Autodesk Inventor part; units mm, degrees
(part 2 of 3)
sketch "Sketch8" plane through (-4.2986, 24.5, 27.7) normal (0, 1, 0) x (1, 0, 0)
  circle A0 centre (15.7486, 17.6859) radius 1.25 projected
  arc A1 (23.4169, 15.4064) -> (22.432, 16.0745) centre (20.1359, 11.63) ccw projected
  arc A2 (22.432, 16.0745) -> (22.5072, 16.4265) centre (15.7486, 17.6859) ccw projected
  arc A3 (22.5072, 16.4265) -> (23.6791, 16.634) centre (22.2271, 21.4212) ccw projected
  arc A4 (23.6791, 16.634) -> (23.7233, 17.0505) centre (15.7486, 17.6859) ccw projected
  arc A5 (23.7233, 17.0505) -> (22.621, 17.4993) centre (21.2992, 12.6745) ccw projected
  arc A6 (22.621, 17.4993) -> (22.6214, 17.8592) centre (15.7486, 17.6859) ccw projected
  arc A7 (22.6214, 17.8592) -> (23.7245, 18.3059) centre (21.3089, 22.6865) ccw projected
  arc A8 (23.7245, 18.3059) -> (23.6811, 18.7224) centre (15.7486, 17.6859) ccw projected
  arc A9 (23.6811, 18.7224) -> (22.5097, 18.9322) centre (22.2198, 13.9381) ccw projected
  arc A10 (22.5097, 18.9322) -> (22.4352, 19.2844) centre (15.7486, 17.6859) ccw projected
  arc A11 (22.4352, 19.2844) -> (23.4213, 19.9506) centre (20.1477, 23.7333) ccw projected
  arc A12 (23.4213, 19.9506) -> (23.2923, 20.3491) centre (15.7486, 17.6859) ccw projected
  arc A13 (23.2923, 20.3491) -> (22.1028, 20.3107) centre (22.8576, 15.3654) ccw projected
  arc A14 (22.1028, 20.3107) -> (21.9567, 20.6397) centre (15.7486, 17.6859) ccw projected
  arc A15 (21.9567, 20.6397) -> (22.7828, 21.4964) centre (18.7942, 24.5158) ccw projected
  arc A16 (22.7828, 21.4964) -> (22.5737, 21.8593) centre (15.7486, 17.6859) ccw projected
  arc A17 (22.5737, 21.8593) -> (21.4182, 21.5745) centre (23.1847, 16.8942) ccw projected
  arc A18 (21.4182, 21.5745) -> (21.2069, 21.8659) centre (15.7486, 17.6859) ccw projected
  arc A19 (21.2069, 21.8659) -> (21.8368, 22.8756) centre (17.3077, 24.9998) ccw projected
  arc A20 (21.8368, 22.8756) -> (21.5569, 23.1871) centre (15.7486, 17.6859) ccw projected
  arc A21 (21.5569, 23.1871) -> (20.4858, 22.6683) centre (23.1868, 18.4576) ccw projected
  arc A22 (20.4858, 22.6683) -> (20.2186, 22.9094) centre (15.7486, 17.6859) ccw projected
  arc A23 (20.2186, 22.9094) -> (20.6248, 24.028) centre (15.753, 25.1641) ccw projected
  arc A24 (20.6248, 24.028) -> (20.2862, 24.2745) centre (15.7486, 17.6859) ccw projected
  arc A25 (20.2862, 24.2745) -> (19.3464, 23.5443) centre (22.8638, 19.9872) ccw projected
  arc A26 (19.3464, 23.5443) -> (19.0349, 23.7246) centre (15.7486, 17.6859) ccw projected
  arc A27 (19.0349, 23.7246) -> (19.1997, 24.9033) centre (14.1981, 25.0016) ccw projected
  arc A28 (19.1997, 24.9033) -> (18.8172, 25.074) centre (15.7486, 17.6859) ccw projected
  arc A29 (18.8172, 25.074) -> (18.0498, 24.1644) centre (22.2299, 21.4163) ccw projected
  arc A30 (18.0498, 24.1644) -> (17.7076, 24.2759) centre (15.7486, 17.6859) ccw projected
  arc A31 (17.7076, 24.2759) -> (17.6237, 25.4631) centre (12.711, 24.5194) ccw projected
  arc A32 (17.6237, 25.4631) -> (17.2141, 25.5505) centre (15.7486, 17.6859) ccw projected
  arc A33 (17.2141, 25.5505) -> (16.6525, 24.5012) centre (21.3127, 22.6823) ccw projected
  arc A34 (16.6525, 24.5012) -> (16.2946, 24.5392) centre (15.7486, 17.6859) ccw projected
  arc A35 (16.2946, 24.5392) -> (15.9657, 25.683) centre (11.3566, 23.7385) ccw projected
  arc A36 (15.9657, 25.683) -> (15.5469, 25.6834) centre (15.7486, 17.6859) ccw projected
  arc A37 (15.5469, 25.6834) -> (15.2158, 24.5402) centre (20.1523, 23.7299) ccw projected
  arc A38 (15.2158, 24.5402) -> (14.8578, 24.503) centre (15.7486, 17.6859) ccw projected
  arc A39 (14.8578, 24.503) -> (14.2983, 25.5534) centre (10.1942, 22.6931) ccw projected
  arc A40 (14.2983, 25.5534) -> (13.8885, 25.4667) centre (15.7486, 17.6859) ccw projected
  arc A41 (13.8885, 25.4667) -> (13.8024, 24.2797) centre (18.7994, 24.5135) ccw projected
  arc A42 (13.8024, 24.2797) -> (13.4599, 24.1688) centre (15.7486, 17.6859) ccw projected
  arc A43 (13.4599, 24.1688) -> (12.6943, 25.0799) centre (9.2745, 21.4288) ccw projected
  arc A44 (12.6943, 25.0799) -> (12.3115, 24.9099) centre (15.7486, 17.6859) ccw projected
  arc A45 (12.3115, 24.9099) -> (12.474, 23.731) centre (17.3132, 24.9986) ccw projected
  arc A46 (12.474, 23.731) -> (12.1621, 23.5513) centre (15.7486, 17.6859) ccw projected
  arc A47 (12.1621, 23.5513) -> (11.2237, 24.2833) centre (8.6378, 20.001) ccw projected
  arc A48 (11.2237, 24.2833) -> (10.8846, 24.0375) centre (15.7486, 17.6859) ccw projected
  arc A49 (10.8846, 24.0375) -> (11.2887, 22.918) centre (15.7587, 25.1641) ccw projected
  arc A50 (11.2887, 22.918) -> (11.021, 22.6775) centre (15.7486, 17.6859) ccw projected
  arc A51 (11.021, 22.6775) -> (9.9509, 23.1984) centre (8.3118, 18.472) ccw projected
  arc A52 (9.9509, 23.1984) -> (9.6704, 22.8874) centre (15.7486, 17.6859) ccw projected
  arc A53 (9.6704, 22.8874) -> (10.2983, 21.8764) centre (14.2036, 25.0028) ccw projected
  arc A54 (10.2983, 21.8764) -> (10.0865, 21.5855) centre (15.7486, 17.6859) ccw projected
  arc A55 (10.0865, 21.5855) -> (8.9315, 21.8725) centre (8.3109, 16.9086) ccw projected
  arc A56 (8.9315, 21.8725) -> (8.7217, 21.51) centre (15.7486, 17.6859) ccw projected
  arc A57 (8.7217, 21.51) -> (9.5462, 20.6517) centre (12.7161, 24.5217) ccw projected
  arc A58 (9.5462, 20.6517) -> (9.3994, 20.323) centre (15.7486, 17.6859) ccw projected
  arc A59 (9.3994, 20.323) -> (8.21, 20.3637) centre (8.635, 15.3792) ccw projected
  arc A60 (8.21, 20.3637) -> (8.0802, 19.9655) centre (15.7486, 17.6859) ccw projected
  arc A61 (8.0802, 19.9655) -> (9.0651, 19.2973) centre (11.3612, 23.7418) ccw projected
  arc A62 (9.0651, 19.2973) -> (8.9899, 18.9453) centre (15.7486, 17.6859) ccw projected
  arc A63 (8.9899, 18.9453) -> (7.818, 18.7378) centre (9.2701, 13.9507) ccw projected
  arc A64 (7.818, 18.7378) -> (7.7738, 18.3213) centre (15.7486, 17.6859) ccw projected
  arc A65 (7.7738, 18.3213) -> (8.8761, 17.8726) centre (10.198, 22.6973) ccw projected
  arc A66 (8.8761, 17.8726) -> (8.8757, 17.5126) centre (15.7486, 17.6859) ccw projected
  arc A67 (8.8757, 17.5126) -> (7.7726, 17.066) centre (10.1882, 12.6853) ccw projected
  arc A68 (7.7726, 17.066) -> (7.816, 16.6494) centre (15.7486, 17.6859) ccw projected
  arc A69 (7.816, 16.6494) -> (8.9875, 16.4396) centre (9.2773, 21.4337) ccw projected
  arc A70 (8.9875, 16.4396) -> (9.062, 16.0875) centre (15.7486, 17.6859) ccw projected
  arc A71 (9.062, 16.0875) -> (8.0758, 15.4212) centre (11.3494, 11.6386) ccw projected
  arc A72 (8.0758, 15.4212) -> (8.2048, 15.0228) centre (15.7486, 17.6859) ccw projected
  arc A73 (8.2048, 15.0228) -> (9.3943, 15.0611) centre (8.6395, 20.0064) ccw projected
  arc A74 (9.3943, 15.0611) -> (9.5404, 14.7322) centre (15.7486, 17.6859) ccw projected
  arc A75 (9.5404, 14.7322) -> (8.7143, 13.8755) centre (12.7029, 10.8561) ccw projected
  arc A76 (8.7143, 13.8755) -> (8.9234, 13.5126) centre (15.7486, 17.6859) ccw projected
  arc A77 (8.9234, 13.5126) -> (10.0789, 13.7974) centre (8.3124, 18.4776) ccw projected
  arc A78 (10.0789, 13.7974) -> (10.2902, 13.506) centre (15.7486, 17.6859) ccw projected
  arc A79 (10.2902, 13.506) -> (9.6603, 12.4962) centre (14.1894, 10.3721) ccw projected
  arc A80 (9.6603, 12.4962) -> (9.9402, 12.1847) centre (15.7486, 17.6859) ccw projected
  arc A81 (9.9402, 12.1847) -> (11.0113, 12.7036) centre (8.3103, 16.9143) ccw projected
  arc A82 (11.0113, 12.7036) -> (11.2785, 12.4625) centre (15.7486, 17.6859) ccw projected
  arc A83 (11.2785, 12.4625) -> (10.8723, 11.3438) centre (15.7441, 10.2078) ccw projected
  arc A84 (10.8723, 11.3438) -> (11.2109, 11.0973) centre (15.7486, 17.6859) ccw projected
  arc A85 (11.2109, 11.0973) -> (12.1507, 11.8275) centre (8.6333, 15.3846) ccw projected
  arc A86 (12.1507, 11.8275) -> (12.4622, 11.6472) centre (15.7486, 17.6859) ccw projected
  arc A87 (12.4622, 11.6472) -> (12.2975, 10.4686) centre (17.299, 10.3702) ccw projected
  arc A88 (12.2975, 10.4686) -> (12.6799, 10.2979) centre (15.7486, 17.6859) ccw projected
  arc A89 (12.6799, 10.2979) -> (13.4474, 11.2075) centre (9.2672, 13.9556) ccw projected
  arc A90 (13.4474, 11.2075) -> (13.7896, 11.0959) centre (15.7486, 17.6859) ccw projected
  arc A91 (13.7896, 11.0959) -> (13.8735, 9.9088) centre (18.7862, 10.8525) ccw projected
  arc A92 (13.8735, 9.9088) -> (14.283, 9.8213) centre (15.7486, 17.6859) ccw projected
  arc A93 (14.283, 9.8213) -> (14.8446, 10.8706) centre (10.1844, 12.6896) ccw projected
  arc A94 (14.8446, 10.8706) -> (15.2025, 10.8326) centre (15.7486, 17.6859) ccw projected
  arc A95 (15.2025, 10.8326) -> (15.5314, 9.6889) centre (20.1405, 11.6334) ccw projected
  arc A96 (15.5314, 9.6889) -> (15.9502, 9.6885) centre (15.7486, 17.6859) ccw projected
  arc A97 (15.9502, 9.6885) -> (16.2813, 10.8316) centre (11.3448, 11.6419) ccw projected
  arc A98 (16.2813, 10.8316) -> (16.6393, 10.8689) centre (15.7486, 17.6859) ccw projected
  arc A99 (16.6393, 10.8689) -> (17.1988, 9.8185) centre (21.303, 12.6788) ccw projected
  arc A100 (17.1988, 9.8185) -> (17.6086, 9.9052) centre (15.7486, 17.6859) ccw projected
  arc A101 (17.6086, 9.9052) -> (17.6948, 11.0921) centre (12.6977, 10.8584) ccw projected
  arc A102 (17.6948, 11.0921) -> (18.0372, 11.203) centre (15.7486, 17.6859) ccw projected
  arc A103 (18.0372, 11.203) -> (18.8029, 10.2919) centre (22.2226, 13.943) ccw projected
  arc A104 (18.8029, 10.2919) -> (19.1856, 10.4619) centre (15.7486, 17.6859) ccw projected
  arc A105 (19.1856, 10.4619) -> (19.0232, 11.6409) centre (14.1839, 10.3733) ccw projected
  arc A106 (19.0232, 11.6409) -> (19.335, 11.8205) centre (15.7486, 17.6859) ccw projected
  arc A107 (19.335, 11.8205) -> (20.2734, 11.0885) centre (22.8594, 15.3708) ccw projected
  arc A108 (20.2734, 11.0885) -> (20.6125, 11.3344) centre (15.7486, 17.6859) ccw projected
  arc A109 (20.6125, 11.3344) -> (20.2084, 12.4538) centre (15.7385, 10.2078) ccw projected
  arc A110 (20.2084, 12.4538) -> (20.4762, 12.6944) centre (15.7486, 17.6859) ccw projected
  arc A111 (20.4762, 12.6944) -> (21.5462, 12.1735) centre (23.1853, 16.8998) ccw projected
  arc A112 (21.5462, 12.1735) -> (21.8268, 12.4844) centre (15.7486, 17.6859) ccw projected
  arc A113 (21.8268, 12.4844) -> (21.1988, 13.4954) centre (17.2935, 10.3691) ccw projected
  arc A114 (21.1988, 13.4954) -> (21.4106, 13.7864) centre (15.7486, 17.6859) ccw projected
  arc A115 (21.4106, 13.7864) -> (22.5656, 13.4993) centre (23.1862, 18.4632) ccw projected
  arc A116 (22.5656, 13.4993) -> (22.7754, 13.8618) centre (15.7486, 17.6859) ccw projected
  arc A117 (22.7754, 13.8618) -> (21.951, 14.7201) centre (18.781, 10.8502) ccw projected
  arc A118 (21.951, 14.7201) -> (22.0977, 15.0488) centre (15.7486, 17.6859) ccw projected
  arc A119 (22.0977, 15.0488) -> (23.2871, 15.0081) centre (22.8621, 19.9926) ccw projected
  arc A120 (23.2871, 15.0081) -> (23.4169, 15.4064) centre (15.7486, 17.6859) ccw projected
  circle A121 centre (15.7486, 17.6859) radius 8
  circle A122 centre (15.7486, 17.6859) radius 8.4
  line L0 (7.6044, 15.6287) -> (7.3834, 15.5214)
  line L1 (31.7444, 20.1683) -> (32.1777, 20.1683) projected
  line L2 (32.1777, 20.1683) -> (35.8615, 24.6355) projected
  line L3 (39.4105, 21.7089) -> (39.4105, 0) projected
  line L4 (39.4105, 0) -> (43.7986, 0) projected
  line L5 (43.7986, 0) -> (43.7986, 27.7) projected
  line L6 (43.7986, 27.7) -> (-10.0014, 27.7) projected
  line L7 (-10.0014, 27.7) -> (-10.0014, 0) projected
  line L8 (-10.0014, 0) -> (0, 0) projected
  arc A123 (0, 0) -> (10.1832, 0) centre (5.0916, 5.5748) ccw projected
  line L9 (10.1832, 0) -> (23.789, 0) projected
  arc A124 (20.8845, 2.8543) -> (23.789, 1) centre (29.9486, 13.85) ccw projected
  line L10 (20.8845, 2.8543) -> (20.8845, 5.5354) projected
  line L11 (24.1705, 10.4583) -> (24.5486, 13.85) projected
  arc A125 (31.7444, 20.1683) -> (27.6265, 18.7253) centre (28.4986, 22.8337) ccw projected
  line L12 (39.4105, 21.7089) -> (39.4105, 0) projected
  line L13 (10.1832, 0) -> (23.789, 0) projected
  line L14 (39.4105, 0) -> (23.789, 0)
  circle A126 centre (28.4986, 22.8337) radius 4.2
  line L15 (23.789, 0) -> (23.789, 1) projected
  arc A127 (20.8845, 5.5354) -> (24.0356, 3.0645) centre (29.9486, 13.85) ccw projected
  line L16 (24.0356, 3.0645) -> (27.7194, 7.5317) projected
  arc A128 (39.4105, 21.7089) -> (35.8615, 24.6355) centre (29.9486, 13.85) ccw projected
  arc A129 (24.1705, 10.4583) -> (27.7194, 7.5317) centre (29.9486, 13.85) ccw projected
  arc A130 (27.6265, 18.7253) -> (24.5486, 13.85) centre (29.9486, 13.85) ccw projected
  point P0 (4.2986, 27.7)
  dimension "d38" = 0.4
  constraints: 4 end point, 2 coincident, 9 other
extrude "Extrusion8" add sketch "Sketch8" along normal blind 2.1 contours A0 | A120 A119 A118 A117 A116 A115 A114 A113 A112 A111 A110 A109 A108 A107 A106 A105 A104 A103 A102 A101 A100 A99 A98 A97 A96 A95 A94 A93 A92 A91 A90 A89 A88 A87 A86 A85 A84 A83 A82 A81 A80 A79 A78 A77 A76 A75 A74 A73 A72 A71 A70 A69 A68 A67 A66 A65 A64 A63 A62 A61 A60 A59 A58 A57 A56 A55 A54 A53 A52 A51 A50 A49 A48 A47 A46 A45 A44 A43 A42 A41 A40 A39 A38 A37 A36 A35 A34 A33 A32 A31 A30 A29 A28 A27 A26 A25 A24 A23 A22 A21 A20 A19 A18 A17 A16 A15 A14 A13 A12 A11 A10 A9 A8 A7 A6 A5 A4 A3 A2 A1 | A1 A2 A3 A121 | A121 A117 A118 A119 | A5 A6 A7 A121 | A121 A113 A114 A115 | A121 A109 A110 A111 | A9 A10 A11 A121 | A121 A105 A106 A107 | A13 A14 A15 A121 | A121 A101 A102 A103 | A17 A18 A19 A121 | A121 A97 A98 A99 | A21 A22 A23 A121 | A121 A93 A94 A95 | A25 A26 A27 A121 | A121 A89 A90 A91 | A29 A30 A31 A121 | A121 A85 A86 A87 | A33 A34 A35 A121 | A121 A81 A82 A83 | A37 A38 A39 A121 | A121 A77 A78 A79 | A41 A42 A43 A121 | A121 A73 A74 A75 | A45 A46 A47 A121 | A121 A69 A70 A71 | A49 A50 A51 A121 | A121 A65 A66 A67 | A53 A54 A55 A121 | A121 A61 A62 A63 | A57 A58 A59 A121 | A122 | A125 A130 L11 A129 L16 A127 L10 A124 L15 L9 A123 L8 L7 L6 L5 L4 L3 A128 L2 L1 | L1 L2 A128 L3 L14 L15 A124 L10 A127 L16 A129 L11 A130 A126
sketch "Sketch10" plane through (-4.2986, 26.6, 27.7) normal (0, 1, 0) x (1, 0, 0)
  line L0 (36.5978, 20.9908) -> (36.5978, 20.9908)
  line L1 (36.5978, 20.9908) -> (36.5978, 20.9908)
  line L2 (43.7986, 0) -> (43.7986, 27.7) projected
  line L3 (43.7986, 0) -> (-14.5322, 0)
  line L4 (43.7986, 0) -> (43.7986, 27.7) projected
  line L5 (43.7986, 27.7) -> (-10.0014, 27.7) projected
  line L6 (-10.0014, 27.7) -> (-10.0014, 0) projected
  line L7 (-10.0014, 0) -> (0, 0) projected
  arc A0 (0, 0) -> (10.1832, 0) centre (5.0916, 5.5748) ccw projected
  circle A1 centre (28.4986, 22.8337) radius 5.5 projected
  circle A2 centre (2.9986, 22.8337) radius 5.5 projected
  circle A3 centre (28.4986, 22.8337) radius 5.9
  circle A4 centre (2.9986, 22.8337) radius 5.9
  line L8 (10.1832, 0) -> (43.7986, 0) projected
  point P0 (4.2986, 27.7)
  dimension "d63" = 0.4
  dimension "d64" = 0.4
  constraints: 6 end point, 3 horizontal, 2 centre point
  measures "d63" radial gap between concentric circles of A1 A3
  measures "d64" radial gap between concentric circles of A2 A4
extrude "Extrusion10" cut sketch "Sketch10" against normal blind 1 contours A3 L5 A1 | L5 A1 A3 | A1 L5 | L5 A1 | A4 L5 A2 | L5 A2 A4 | A2 L5 | L5 A2
sketch "Sketch11" plane through (-4.2986, 25.6, 27.7) normal (0, 1, 0) x (1, 0, 0)
  circle A0 centre (28.4986, 22.8337) radius 3 projected
  arc A1 (18.0491, 21.8046) -> (19.212, 21.5492) centre (19.8204, 27.0964) ccw projected
  arc A2 (19.212, 21.5492) -> (19.2696, 21.1856) centre (28.4986, 22.8337) ccw projected
  arc A3 (19.2696, 21.1856) -> (18.2425, 20.5835) centre (21.5624, 16.098) ccw projected
  arc A4 (18.2425, 20.5835) -> (18.3388, 20.1826) centre (28.4986, 22.8337) ccw projected
  arc A5 (18.3388, 20.1826) -> (19.5272, 20.1123) centre (19.2604, 25.6863) ccw projected
  arc A6 (19.5272, 20.1123) -> (19.641, 19.7622) centre (28.4986, 22.8337) ccw projected
  arc A7 (19.641, 19.7622) -> (18.7208, 19.0068) centre (22.7015, 15.0959) ccw projected
  arc A8 (18.7208, 19.0068) -> (18.8786, 18.6259) centre (28.4986, 22.8337) ccw projected
  arc A9 (18.8786, 18.6259) -> (20.0634, 18.7424) centre (18.9279, 24.2061) ccw projected
  arc A10 (20.0634, 18.7424) -> (20.2305, 18.4144) centre (28.4986, 22.8337) ccw projected
  arc A11 (20.2305, 18.4144) -> (19.4399, 17.5243) centre (23.9833, 14.2843) ccw projected
  arc A12 (19.4399, 17.5243) -> (19.6553, 17.1728) centre (28.4986, 22.8337) ccw projected
  arc A13 (19.6553, 17.1728) -> (20.8073, 17.4732) centre (18.8311, 22.692) ccw projected
  arc A14 (20.8073, 17.4732) -> (21.0237, 17.1754) centre (28.4986, 22.8337) ccw projected
  arc A15 (21.0237, 17.1754) -> (20.382, 16.1726) centre (25.3763, 13.6832) ccw projected
  arc A16 (20.382, 16.1726) -> (20.6497, 15.8591) centre (28.4986, 22.8337) ccw projected
  arc A17 (20.6497, 15.8591) -> (21.7406, 16.336) centre (18.9723, 21.1814) ccw projected
  arc A18 (21.7406, 16.336) -> (22.0009, 16.0757) centre (28.4986, 22.8337) ccw projected
  arc A19 (22.0009, 16.0757) -> (21.5239, 14.9849) centre (26.8462, 13.3075) ccw projected
  arc A20 (21.5239, 14.9849) -> (21.8374, 14.7171) centre (28.4986, 22.8337) ccw projected
  arc A21 (21.8374, 14.7171) -> (22.8402, 15.3589) centre (19.3481, 19.7115) ccw projected
  arc A22 (22.8402, 15.3589) -> (23.138, 15.1425) centre (28.4986, 22.8337) ccw projected
  arc A23 (23.138, 15.1425) -> (22.8376, 13.9905) centre (28.3568, 13.1663) ccw projected
  arc A24 (22.8376, 13.9905) -> (23.1892, 13.775) centre (28.4986, 22.8337) ccw projected
  arc A25 (23.1892, 13.775) -> (24.0792, 14.5657) centre (19.9491, 18.3185) ccw projected
  arc A26 (24.0792, 14.5657) -> (24.4072, 14.3986) centre (28.4986, 22.8337) ccw projected
  arc A27 (24.4072, 14.3986) -> (24.2907, 13.2138) centre (29.8709, 13.2631) ccw projected
  arc A28 (24.2907, 13.2138) -> (24.6716, 13.056) centre (28.4986, 22.8337) ccw projected
  arc A29 (24.6716, 13.056) -> (25.427, 13.9762) centre (20.7607, 17.0367) ccw projected
  arc A30 (25.427, 13.9762) -> (25.7771, 13.8624) centre (28.4986, 22.8337) ccw projected
  arc A31 (25.7771, 13.8624) -> (25.8474, 12.6739) centre (31.3512, 13.5956) ccw projected
  arc A32 (25.8474, 12.6739) -> (26.2483, 12.5777) centre (28.4986, 22.8337) ccw projected
  arc A33 (26.2483, 12.5777) -> (26.8505, 13.6047) centre (21.7629, 15.8976) ccw projected
  arc A34 (26.8505, 13.6047) -> (27.2141, 13.5471) centre (28.4986, 22.8337) ccw projected
  arc A35 (27.2141, 13.5471) -> (27.4694, 12.3843) centre (32.7612, 14.1556) ccw projected
  arc A36 (27.4694, 12.3843) -> (27.8804, 12.3519) centre (28.4986, 22.8337) ccw projected
  arc A37 (27.8804, 12.3519) -> (28.3145, 13.4605) centre (22.9308, 14.9293) ccw projected
  arc A38 (28.3145, 13.4605) -> (28.6826, 13.4605) centre (28.4986, 22.8337) ccw projected
  arc A39 (28.6826, 13.4605) -> (29.1167, 12.3519) centre (34.0663, 14.9293) ccw projected
  arc A40 (29.1167, 12.3519) -> (29.5277, 12.3843) centre (28.4986, 22.8337) ccw projected
  arc A41 (29.5277, 12.3843) -> (29.7831, 13.5471) centre (24.2359, 14.1556) ccw projected
  arc A42 (29.7831, 13.5471) -> (30.1467, 13.6047) centre (28.4986, 22.8337) ccw projected
  arc A43 (30.1467, 13.6047) -> (30.7488, 12.5777) centre (35.2343, 15.8976) ccw projected
  arc A44 (30.7488, 12.5777) -> (31.1497, 12.6739) centre (28.4986, 22.8337) ccw projected
  arc A45 (31.1497, 12.6739) -> (31.22, 13.8624) centre (25.646, 13.5956) ccw projected
  arc A46 (31.22, 13.8624) -> (31.5701, 13.9762) centre (28.4986, 22.8337) ccw projected
  arc A47 (31.5701, 13.9762) -> (32.3255, 13.056) centre (36.2364, 17.0367) ccw projected
  arc A48 (32.3255, 13.056) -> (32.7064, 13.2138) centre (28.4986, 22.8337) ccw projected
  arc A49 (32.7064, 13.2138) -> (32.5899, 14.3986) centre (27.1262, 13.2631) ccw projected
  arc A50 (32.5899, 14.3986) -> (32.9179, 14.5657) centre (28.4986, 22.8337) ccw projected
  arc A51 (32.9179, 14.5657) -> (33.808, 13.775) centre (37.048, 18.3185) ccw projected
  arc A52 (33.808, 13.775) -> (34.1595, 13.9905) centre (28.4986, 22.8337) ccw projected
  arc A53 (34.1595, 13.9905) -> (33.8591, 15.1425) centre (28.6403, 13.1663) ccw projected
  arc A54 (33.8591, 15.1425) -> (34.1569, 15.3589) centre (28.4986, 22.8337) ccw projected
  arc A55 (34.1569, 15.3589) -> (35.1597, 14.7171) centre (37.6491, 19.7115) ccw projected
  arc A56 (35.1597, 14.7171) -> (35.4732, 14.9849) centre (28.4986, 22.8337) ccw projected
  arc A57 (35.4732, 14.9849) -> (34.9963, 16.0757) centre (30.1509, 13.3075) ccw projected
  arc A58 (34.9963, 16.0757) -> (35.2566, 16.336) centre (28.4986, 22.8337) ccw projected
  arc A59 (35.2566, 16.336) -> (36.3474, 15.8591) centre (38.0248, 21.1814) ccw projected
  arc A60 (36.3474, 15.8591) -> (36.6152, 16.1726) centre (28.4986, 22.8337) ccw projected
  arc A61 (36.6152, 16.1726) -> (35.9734, 17.1754) centre (31.6208, 13.6832) ccw projected
  arc A62 (35.9734, 17.1754) -> (36.1898, 17.4732) centre (28.4986, 22.8337) ccw projected
  arc A63 (36.1898, 17.4732) -> (37.3418, 17.1728) centre (38.166, 22.692) ccw projected
  arc A64 (37.3418, 17.1728) -> (37.5573, 17.5243) centre (28.4986, 22.8337) ccw projected
  arc A65 (37.5573, 17.5243) -> (36.7666, 18.4144) centre (33.0138, 14.2843) ccw projected
  arc A66 (36.7666, 18.4144) -> (36.9337, 18.7424) centre (28.4986, 22.8337) ccw projected
  arc A67 (36.9337, 18.7424) -> (38.1185, 18.6259) centre (38.0692, 24.2061) ccw projected
  arc A68 (38.1185, 18.6259) -> (38.2763, 19.0068) centre (28.4986, 22.8337) ccw projected
  arc A69 (38.2763, 19.0068) -> (37.3561, 19.7622) centre (34.2956, 15.0959) ccw projected
  arc A70 (37.3561, 19.7622) -> (37.4699, 20.1123) centre (28.4986, 22.8337) ccw projected
  arc A71 (37.4699, 20.1123) -> (38.6584, 20.1826) centre (37.7367, 25.6863) ccw projected
  arc A72 (38.6584, 20.1826) -> (38.7546, 20.5835) centre (28.4986, 22.8337) ccw projected
  arc A73 (38.7546, 20.5835) -> (37.7276, 21.1856) centre (35.4347, 16.098) ccw projected
  arc A74 (37.7276, 21.1856) -> (37.7851, 21.5492) centre (28.4986, 22.8337) ccw projected
  arc A75 (37.7851, 21.5492) -> (38.948, 21.8046) centre (37.1767, 27.0964) ccw projected
  arc A76 (38.948, 21.8046) -> (38.9804, 22.2156) centre (28.4986, 22.8337) ccw projected
  arc A77 (38.9804, 22.2156) -> (37.8718, 22.6497) centre (36.403, 17.266) ccw projected
  arc A78 (37.8718, 22.6497) -> (37.8718, 23.0178) centre (28.4986, 22.8337) ccw projected
  arc A79 (37.8718, 23.0178) -> (38.9804, 23.4519) centre (36.403, 28.4015) ccw projected
  arc A80 (38.9804, 23.4519) -> (38.948, 23.8629) centre (28.4986, 22.8337) ccw projected
  arc A81 (38.948, 23.8629) -> (37.7851, 24.1182) centre (37.1767, 18.5711) ccw projected
  arc A82 (37.7851, 24.1182) -> (37.7276, 24.4818) centre (28.4986, 22.8337) ccw projected
  arc A83 (37.7276, 24.4818) -> (38.7546, 25.084) centre (35.4347, 29.5694) ccw projected
  arc A84 (38.7546, 25.084) -> (38.6584, 25.4849) centre (28.4986, 22.8337) ccw projected
  arc A85 (38.6584, 25.4849) -> (37.4699, 25.5552) centre (37.7367, 19.9811) ccw projected
  arc A86 (37.4699, 25.5552) -> (37.3561, 25.9053) centre (28.4986, 22.8337) ccw projected
  arc A87 (37.3561, 25.9053) -> (38.2763, 26.6607) centre (34.2956, 30.5716) ccw projected
  arc A88 (38.2763, 26.6607) -> (38.1185, 27.0416) centre (28.4986, 22.8337) ccw projected
  arc A89 (38.1185, 27.0416) -> (36.9337, 26.9251) centre (38.0692, 21.4614) ccw projected
  arc A90 (36.9337, 26.9251) -> (36.7666, 27.2531) centre (28.4986, 22.8337) ccw projected
  arc A91 (36.7666, 27.2531) -> (37.5573, 28.1431) centre (33.0138, 31.3832) ccw projected
  arc A92 (37.5573, 28.1431) -> (37.3418, 28.4947) centre (28.4986, 22.8337) ccw projected
  arc A93 (37.3418, 28.4947) -> (36.1898, 28.1942) centre (38.166, 22.9755) ccw projected
  arc A94 (36.1898, 28.1942) -> (35.9734, 28.4921) centre (28.4986, 22.8337) ccw projected
  arc A95 (35.9734, 28.4921) -> (36.6152, 29.4949) centre (31.6208, 31.9842) ccw projected
  arc A96 (36.6152, 29.4949) -> (36.3474, 29.8084) centre (28.4986, 22.8337) ccw projected
  arc A97 (36.3474, 29.8084) -> (35.2566, 29.3314) centre (38.0248, 24.4861) ccw projected
  arc A98 (35.2566, 29.3314) -> (34.9963, 29.5917) centre (28.4986, 22.8337) ccw projected
  arc A99 (34.9963, 29.5917) -> (35.4732, 30.6826) centre (30.1509, 32.36) ccw projected
  arc A100 (35.4732, 30.6826) -> (35.1597, 30.9503) centre (28.4986, 22.8337) ccw projected
  arc A101 (35.1597, 30.9503) -> (34.1569, 30.3086) centre (37.6491, 25.956) ccw projected
  arc A102 (34.1569, 30.3086) -> (33.8591, 30.525) centre (28.4986, 22.8337) ccw projected
  arc A103 (33.8591, 30.525) -> (34.1595, 31.677) centre (28.6403, 32.5012) ccw projected
  arc A104 (34.1595, 31.677) -> (33.808, 31.8924) centre (28.4986, 22.8337) ccw projected
  arc A105 (33.808, 31.8924) -> (32.9179, 31.1017) centre (37.048, 27.349) ccw projected
  arc A106 (32.9179, 31.1017) -> (32.5899, 31.2689) centre (28.4986, 22.8337) ccw projected
  arc A107 (32.5899, 31.2689) -> (32.7064, 32.4537) centre (27.1262, 32.4044) ccw projected
  arc A108 (32.7064, 32.4537) -> (32.3255, 32.6115) centre (28.4986, 22.8337) ccw projected
  arc A109 (32.3255, 32.6115) -> (31.5701, 31.6913) centre (36.2364, 28.6308) ccw projected
  arc A110 (31.5701, 31.6913) -> (31.22, 31.8051) centre (28.4986, 22.8337) ccw projected
  arc A111 (31.22, 31.8051) -> (31.1497, 32.9935) centre (25.646, 32.0719) ccw projected
  arc A112 (31.1497, 32.9935) -> (30.7488, 33.0898) centre (28.4986, 22.8337) ccw projected
  arc A113 (30.7488, 33.0898) -> (30.1467, 32.0627) centre (35.2343, 29.7699) ccw projected
  arc A114 (30.1467, 32.0627) -> (29.7831, 32.1203) centre (28.4986, 22.8337) ccw projected
  arc A115 (29.7831, 32.1203) -> (29.5277, 33.2832) centre (24.2359, 31.5119) ccw projected
  arc A116 (29.5277, 33.2832) -> (29.1167, 33.3155) centre (28.4986, 22.8337) ccw projected
  arc A117 (29.1167, 33.3155) -> (28.6826, 32.2069) centre (34.0663, 30.7382) ccw projected
  arc A118 (28.6826, 32.2069) -> (28.3145, 32.2069) centre (28.4986, 22.8337) ccw projected
  arc A119 (28.3145, 32.2069) -> (27.8804, 33.3155) centre (22.9308, 30.7382) ccw projected
  arc A120 (27.8804, 33.3155) -> (27.4694, 33.2832) centre (28.4986, 22.8337) ccw projected
  arc A121 (27.4694, 33.2832) -> (27.2141, 32.1203) centre (32.7612, 31.5119) ccw projected
  arc A122 (27.2141, 32.1203) -> (26.8505, 32.0627) centre (28.4986, 22.8337) ccw projected
  arc A123 (26.8505, 32.0627) -> (26.2483, 33.0898) centre (21.7629, 29.7699) ccw projected
  arc A124 (26.2483, 33.0898) -> (25.8474, 32.9935) centre (28.4986, 22.8337) ccw projected
  arc A125 (25.8474, 32.9935) -> (25.7771, 31.8051) centre (31.3512, 32.0719) ccw projected
  arc A126 (25.7771, 31.8051) -> (25.427, 31.6913) centre (28.4986, 22.8337) ccw projected
  arc A127 (25.427, 31.6913) -> (24.6716, 32.6115) centre (20.7607, 28.6308) ccw projected
  arc A128 (24.6716, 32.6115) -> (24.2907, 32.4537) centre (28.4986, 22.8337) ccw projected
  arc A129 (24.2907, 32.4537) -> (24.4072, 31.2689) centre (29.8709, 32.4044) ccw projected
  arc A130 (24.4072, 31.2689) -> (24.0792, 31.1017) centre (28.4986, 22.8337) ccw projected
  arc A131 (24.0792, 31.1017) -> (23.1892, 31.8924) centre (19.9491, 27.349) ccw projected
  arc A132 (23.1892, 31.8924) -> (22.8376, 31.677) centre (28.4986, 22.8337) ccw projected
  arc A133 (22.8376, 31.677) -> (23.138, 30.525) centre (28.3568, 32.5012) ccw projected
  arc A134 (23.138, 30.525) -> (22.8402, 30.3086) centre (28.4986, 22.8337) ccw projected
  arc A135 (22.8402, 30.3086) -> (21.8374, 30.9503) centre (19.3481, 25.956) ccw projected
  arc A136 (21.8374, 30.9503) -> (21.5239, 30.6826) centre (28.4986, 22.8337) ccw projected
  arc A137 (21.5239, 30.6826) -> (22.0009, 29.5917) centre (26.8462, 32.36) ccw projected
  arc A138 (22.0009, 29.5917) -> (21.7406, 29.3314) centre (28.4986, 22.8337) ccw projected
  arc A139 (21.7406, 29.3314) -> (20.6497, 29.8084) centre (18.9723, 24.4861) ccw projected
  arc A140 (20.6497, 29.8084) -> (20.382, 29.4949) centre (28.4986, 22.8337) ccw projected
  arc A141 (20.382, 29.4949) -> (21.0237, 28.4921) centre (25.3763, 31.9842) ccw projected
  arc A142 (21.0237, 28.4921) -> (20.8073, 28.1942) centre (28.4986, 22.8337) ccw projected
  arc A143 (20.8073, 28.1942) -> (19.6553, 28.4947) centre (18.8311, 22.9755) ccw projected
  arc A144 (19.6553, 28.4947) -> (19.4399, 28.1431) centre (28.4986, 22.8337) ccw projected
  arc A145 (19.4399, 28.1431) -> (20.2305, 27.2531) centre (23.9833, 31.3832) ccw projected
  arc A146 (20.2305, 27.2531) -> (20.0634, 26.9251) centre (28.4986, 22.8337) ccw projected
  arc A147 (20.0634, 26.9251) -> (18.8786, 27.0416) centre (18.9279, 21.4614) ccw projected
  arc A148 (18.8786, 27.0416) -> (18.7208, 26.6607) centre (28.4986, 22.8337) ccw projected
  arc A149 (18.7208, 26.6607) -> (19.641, 25.9053) centre (22.7015, 30.5716) ccw projected
  arc A150 (19.641, 25.9053) -> (19.5272, 25.5552) centre (28.4986, 22.8337) ccw projected
  arc A151 (19.5272, 25.5552) -> (18.3388, 25.4849) centre (19.2604, 19.9811) ccw projected
  arc A152 (18.3388, 25.4849) -> (18.2425, 25.084) centre (28.4986, 22.8337) ccw projected
  arc A153 (18.2425, 25.084) -> (19.2696, 24.4818) centre (21.5624, 29.5694) ccw projected
  arc A154 (19.2696, 24.4818) -> (19.212, 24.1182) centre (28.4986, 22.8337) ccw projected
  arc A155 (19.212, 24.1182) -> (18.0491, 23.8629) centre (19.8204, 18.5711) ccw projected
  arc A156 (18.0491, 23.8629) -> (18.0168, 23.4519) centre (28.4986, 22.8337) ccw projected
  arc A157 (18.0168, 23.4519) -> (19.1254, 23.0178) centre (20.5941, 28.4015) ccw projected
  arc A158 (19.1254, 23.0178) -> (19.1254, 22.6497) centre (28.4986, 22.8337) ccw projected
  arc A159 (19.1254, 22.6497) -> (18.0168, 22.2156) centre (20.5941, 17.266) ccw projected
  arc A160 (18.0168, 22.2156) -> (18.0491, 21.8046) centre (28.4986, 22.8337) ccw projected
  circle A161 centre (2.9986, 22.8337) radius 3 projected
  arc A162 (13.448, 23.8629) -> (12.2851, 24.1182) centre (11.6767, 18.5711) ccw projected
  arc A163 (12.2851, 24.1182) -> (12.2276, 24.4818) centre (2.9986, 22.8337) ccw projected
  arc A164 (12.2276, 24.4818) -> (13.2546, 25.084) centre (9.9347, 29.5694) ccw projected
  arc A165 (13.2546, 25.084) -> (13.1584, 25.4849) centre (2.9986, 22.8337) ccw projected
  arc A166 (13.1584, 25.4849) -> (11.9699, 25.5552) centre (12.2367, 19.9811) ccw projected
  arc A167 (11.9699, 25.5552) -> (11.8561, 25.9053) centre (2.9986, 22.8337) ccw projected
  arc A168 (11.8561, 25.9053) -> (12.7763, 26.6607) centre (8.7956, 30.5716) ccw projected
  arc A169 (12.7763, 26.6607) -> (12.6185, 27.0416) centre (2.9986, 22.8337) ccw projected
  arc A170 (12.6185, 27.0416) -> (11.4337, 26.9251) centre (12.5692, 21.4614) ccw projected
  arc A171 (11.4337, 26.9251) -> (11.2666, 27.2531) centre (2.9986, 22.8337) ccw projected
  arc A172 (11.2666, 27.2531) -> (12.0573, 28.1431) centre (7.5138, 31.3832) ccw projected
  arc A173 (12.0573, 28.1431) -> (11.8418, 28.4947) centre (2.9986, 22.8337) ccw projected
  arc A174 (11.8418, 28.4947) -> (10.6898, 28.1942) centre (12.666, 22.9755) ccw projected
  arc A175 (10.6898, 28.1942) -> (10.4734, 28.4921) centre (2.9986, 22.8337) ccw projected
  arc A176 (10.4734, 28.4921) -> (11.1152, 29.4949) centre (6.1208, 31.9842) ccw projected
  arc A177 (11.1152, 29.4949) -> (10.8474, 29.8084) centre (2.9986, 22.8337) ccw projected
  arc A178 (10.8474, 29.8084) -> (9.7566, 29.3314) centre (12.5248, 24.4861) ccw projected
  arc A179 (9.7566, 29.3314) -> (9.4963, 29.5917) centre (2.9986, 22.8337) ccw projected
  arc A180 (9.4963, 29.5917) -> (9.9732, 30.6826) centre (4.6509, 32.36) ccw projected
  arc A181 (9.9732, 30.6826) -> (9.6597, 30.9503) centre (2.9986, 22.8337) ccw projected
  arc A182 (9.6597, 30.9503) -> (8.6569, 30.3086) centre (12.1491, 25.956) ccw projected
  arc A183 (8.6569, 30.3086) -> (8.3591, 30.525) centre (2.9986, 22.8337) ccw projected
  arc A184 (8.3591, 30.525) -> (8.6595, 31.677) centre (3.1403, 32.5012) ccw projected
  arc A185 (8.6595, 31.677) -> (8.308, 31.8924) centre (2.9986, 22.8337) ccw projected
  arc A186 (8.308, 31.8924) -> (7.4179, 31.1017) centre (11.548, 27.349) ccw projected
  arc A187 (7.4179, 31.1017) -> (7.0899, 31.2689) centre (2.9986, 22.8337) ccw projected
  arc A188 (7.0899, 31.2689) -> (7.2064, 32.4537) centre (1.6262, 32.4044) ccw projected
  arc A189 (7.2064, 32.4537) -> (6.8255, 32.6115) centre (2.9986, 22.8337) ccw projected
  arc A190 (6.8255, 32.6115) -> (6.0701, 31.6913) centre (10.7364, 28.6308) ccw projected
  arc A191 (6.0701, 31.6913) -> (5.72, 31.8051) centre (2.9986, 22.8337) ccw projected
  arc A192 (5.72, 31.8051) -> (5.6497, 32.9935) centre (0.146, 32.0719) ccw projected
  arc A193 (5.6497, 32.9935) -> (5.2488, 33.0898) centre (2.9986, 22.8337) ccw projected
  arc A194 (5.2488, 33.0898) -> (4.6467, 32.0627) centre (9.7343, 29.7699) ccw projected
  arc A195 (4.6467, 32.0627) -> (4.2831, 32.1203) centre (2.9986, 22.8337) ccw projected
  arc A196 (4.2831, 32.1203) -> (4.0277, 33.2832) centre (-1.2641, 31.5119) ccw projected
  arc A197 (4.0277, 33.2832) -> (3.6167, 33.3155) centre (2.9986, 22.8337) ccw projected
  arc A198 (3.6167, 33.3155) -> (3.1826, 32.2069) centre (8.5663, 30.7382) ccw projected
  arc A199 (3.1826, 32.2069) -> (2.8145, 32.2069) centre (2.9986, 22.8337) ccw projected
  arc A200 (2.8145, 32.2069) -> (2.3804, 33.3155) centre (-2.5692, 30.7382) ccw projected
  arc A201 (2.3804, 33.3155) -> (1.9694, 33.2832) centre (2.9986, 22.8337) ccw projected
  arc A202 (1.9694, 33.2832) -> (1.7141, 32.1203) centre (7.2612, 31.5119) ccw projected
  arc A203 (1.7141, 32.1203) -> (1.3505, 32.0627) centre (2.9986, 22.8337) ccw projected
  arc A204 (1.3505, 32.0627) -> (0.7483, 33.0898) centre (-3.7371, 29.7699) ccw projected
  arc A205 (0.7483, 33.0898) -> (0.3474, 32.9935) centre (2.9986, 22.8337) ccw projected
  arc A206 (0.3474, 32.9935) -> (0.2771, 31.8051) centre (5.8512, 32.0719) ccw projected
  arc A207 (0.2771, 31.8051) -> (-0.073, 31.6913) centre (2.9986, 22.8337) ccw projected
  arc A208 (-0.073, 31.6913) -> (-0.8284, 32.6115) centre (-4.7393, 28.6308) ccw projected
  arc A209 (-0.8284, 32.6115) -> (-1.2093, 32.4537) centre (2.9986, 22.8337) ccw projected
  arc A210 (-1.2093, 32.4537) -> (-1.0928, 31.2689) centre (4.3709, 32.4044) ccw projected
  arc A211 (-1.0928, 31.2689) -> (-1.4208, 31.1017) centre (2.9986, 22.8337) ccw projected
  arc A212 (-1.4208, 31.1017) -> (-2.3108, 31.8924) centre (-5.5509, 27.349) ccw projected
  arc A213 (-2.3108, 31.8924) -> (-2.6624, 31.677) centre (2.9986, 22.8337) ccw projected
  arc A214 (-2.6624, 31.677) -> (-2.362, 30.525) centre (2.8568, 32.5012) ccw projected
  arc A215 (-2.362, 30.525) -> (-2.6598, 30.3086) centre (2.9986, 22.8337) ccw projected
  arc A216 (-2.6598, 30.3086) -> (-3.6626, 30.9503) centre (-6.1519, 25.956) ccw projected
  arc A217 (-3.6626, 30.9503) -> (-3.9761, 30.6826) centre (2.9986, 22.8337) ccw projected
  arc A218 (-3.9761, 30.6826) -> (-3.4991, 29.5917) centre (1.3462, 32.36) ccw projected
  arc A219 (-3.4991, 29.5917) -> (-3.7594, 29.3314) centre (2.9986, 22.8337) ccw projected
  arc A220 (-3.7594, 29.3314) -> (-4.8503, 29.8084) centre (-6.5277, 24.4861) ccw projected
  arc A221 (-4.8503, 29.8084) -> (-5.118, 29.4949) centre (2.9986, 22.8337) ccw projected
  arc A222 (-5.118, 29.4949) -> (-4.4763, 28.4921) centre (-0.1237, 31.9842) ccw projected
  arc A223 (-4.4763, 28.4921) -> (-4.6927, 28.1942) centre (2.9986, 22.8337) ccw projected
  arc A224 (-4.6927, 28.1942) -> (-5.8447, 28.4947) centre (-6.6689, 22.9755) ccw projected
  arc A225 (-5.8447, 28.4947) -> (-6.0601, 28.1431) centre (2.9986, 22.8337) ccw projected
  arc A226 (-6.0601, 28.1431) -> (-5.2695, 27.2531) centre (-1.5167, 31.3832) ccw projected
  arc A227 (-5.2695, 27.2531) -> (-5.4366, 26.9251) centre (2.9986, 22.8337) ccw projected
  arc A228 (-5.4366, 26.9251) -> (-6.6214, 27.0416) centre (-6.5721, 21.4614) ccw projected
  arc A229 (-6.6214, 27.0416) -> (-6.7792, 26.6607) centre (2.9986, 22.8337) ccw projected
  arc A230 (-6.7792, 26.6607) -> (-5.859, 25.9053) centre (-2.7985, 30.5716) ccw projected
  arc A231 (-5.859, 25.9053) -> (-5.9728, 25.5552) centre (2.9986, 22.8337) ccw projected
  arc A232 (-5.9728, 25.5552) -> (-7.1612, 25.4849) centre (-6.2396, 19.9811) ccw projected
  arc A233 (-7.1612, 25.4849) -> (-7.2575, 25.084) centre (2.9986, 22.8337) ccw projected
  arc A234 (-7.2575, 25.084) -> (-6.2304, 24.4818) centre (-3.9376, 29.5694) ccw projected
  arc A235 (-6.2304, 24.4818) -> (-6.288, 24.1182) centre (2.9986, 22.8337) ccw projected
  arc A236 (-6.288, 24.1182) -> (-7.4509, 23.8629) centre (-5.6796, 18.5711) ccw projected
  arc A237 (-7.4509, 23.8629) -> (-7.4832, 23.4519) centre (2.9986, 22.8337) ccw projected
  arc A238 (-7.4832, 23.4519) -> (-6.3746, 23.0178) centre (-4.9059, 28.4015) ccw projected
  arc A239 (-6.3746, 23.0178) -> (-6.3746, 22.6497) centre (2.9986, 22.8337) ccw projected
  arc A240 (-6.3746, 22.6497) -> (-7.4832, 22.2156) centre (-4.9059, 17.266) ccw projected
  arc A241 (-7.4832, 22.2156) -> (-7.4509, 21.8046) centre (2.9986, 22.8337) ccw projected
  arc A242 (-7.4509, 21.8046) -> (-6.288, 21.5492) centre (-5.6796, 27.0964) ccw projected
  arc A243 (-6.288, 21.5492) -> (-6.2304, 21.1856) centre (2.9986, 22.8337) ccw projected
  arc A244 (-6.2304, 21.1856) -> (-7.2575, 20.5835) centre (-3.9376, 16.098) ccw projected
  arc A245 (-7.2575, 20.5835) -> (-7.1612, 20.1826) centre (2.9986, 22.8337) ccw projected
  arc A246 (-7.1612, 20.1826) -> (-5.9728, 20.1123) centre (-6.2396, 25.6863) ccw projected
  arc A247 (-5.9728, 20.1123) -> (-5.859, 19.7622) centre (2.9986, 22.8337) ccw projected
  arc A248 (-5.859, 19.7622) -> (-6.7792, 19.0068) centre (-2.7985, 15.0959) ccw projected
  arc A249 (-6.7792, 19.0068) -> (-6.6214, 18.6259) centre (2.9986, 22.8337) ccw projected
  arc A250 (-6.6214, 18.6259) -> (-5.4366, 18.7424) centre (-6.5721, 24.2061) ccw projected
  arc A251 (-5.4366, 18.7424) -> (-5.2695, 18.4144) centre (2.9986, 22.8337) ccw projected
  arc A252 (-5.2695, 18.4144) -> (-6.0601, 17.5243) centre (-1.5167, 14.2843) ccw projected
  arc A253 (-6.0601, 17.5243) -> (-5.8447, 17.1728) centre (2.9986, 22.8337) ccw projected
  arc A254 (-5.8447, 17.1728) -> (-4.6927, 17.4732) centre (-6.6689, 22.692) ccw projected
  arc A255 (-4.6927, 17.4732) -> (-4.4763, 17.1754) centre (2.9986, 22.8337) ccw projected
  arc A256 (-4.4763, 17.1754) -> (-5.118, 16.1726) centre (-0.1237, 13.6832) ccw projected
  arc A257 (-5.118, 16.1726) -> (-4.8503, 15.8591) centre (2.9986, 22.8337) ccw projected
  arc A258 (-4.8503, 15.8591) -> (-3.7594, 16.336) centre (-6.5277, 21.1814) ccw projected
  arc A259 (-3.7594, 16.336) -> (-3.4991, 16.0757) centre (2.9986, 22.8337) ccw projected
  arc A260 (-3.4991, 16.0757) -> (-3.9761, 14.9849) centre (1.3462, 13.3075) ccw projected
  arc A261 (-3.9761, 14.9849) -> (-3.6626, 14.7171) centre (2.9986, 22.8337) ccw projected
  arc A262 (-3.6626, 14.7171) -> (-2.6598, 15.3589) centre (-6.1519, 19.7115) ccw projected
  arc A263 (-2.6598, 15.3589) -> (-2.362, 15.1425) centre (2.9986, 22.8337) ccw projected
  arc A264 (-2.362, 15.1425) -> (-2.6624, 13.9905) centre (2.8568, 13.1663) ccw projected
  arc A265 (-2.6624, 13.9905) -> (-2.3108, 13.775) centre (2.9986, 22.8337) ccw projected
  arc A266 (-2.3108, 13.775) -> (-1.4208, 14.5657) centre (-5.5509, 18.3185) ccw projected
  arc A267 (-1.4208, 14.5657) -> (-1.0928, 14.3986) centre (2.9986, 22.8337) ccw projected
  arc A268 (-1.0928, 14.3986) -> (-1.2093, 13.2138) centre (4.3709, 13.2631) ccw projected
  arc A269 (-1.2093, 13.2138) -> (-0.8284, 13.056) centre (2.9986, 22.8337) ccw projected
  arc A270 (-0.8284, 13.056) -> (-0.073, 13.9762) centre (-4.7393, 17.0367) ccw projected
  arc A271 (-0.073, 13.9762) -> (0.2771, 13.8624) centre (2.9986, 22.8337) ccw projected
  arc A272 (0.2771, 13.8624) -> (0.3474, 12.6739) centre (5.8512, 13.5956) ccw projected
  arc A273 (0.3474, 12.6739) -> (0.7483, 12.5777) centre (2.9986, 22.8337) ccw projected
  arc A274 (0.7483, 12.5777) -> (1.3505, 13.6047) centre (-3.7371, 15.8976) ccw projected
  arc A275 (1.3505, 13.6047) -> (1.7141, 13.5471) centre (2.9986, 22.8337) ccw projected
  arc A276 (1.7141, 13.5471) -> (1.9694, 12.3843) centre (7.2612, 14.1556) ccw projected
  arc A277 (1.9694, 12.3843) -> (2.3804, 12.3519) centre (2.9986, 22.8337) ccw projected
  arc A278 (2.3804, 12.3519) -> (2.8145, 13.4605) centre (-2.5692, 14.9293) ccw projected
  arc A279 (2.8145, 13.4605) -> (3.1826, 13.4605) centre (2.9986, 22.8337) ccw projected
  arc A280 (3.1826, 13.4605) -> (3.6167, 12.3519) centre (8.5663, 14.9293) ccw projected
  arc A281 (3.6167, 12.3519) -> (4.0277, 12.3843) centre (2.9986, 22.8337) ccw projected
  arc A282 (4.0277, 12.3843) -> (4.2831, 13.5471) centre (-1.2641, 14.1556) ccw projected
  arc A283 (4.2831, 13.5471) -> (4.6467, 13.6047) centre (2.9986, 22.8337) ccw projected
  arc A284 (4.6467, 13.6047) -> (5.2488, 12.5777) centre (9.7343, 15.8976) ccw projected
  arc A285 (5.2488, 12.5777) -> (5.6497, 12.6739) centre (2.9986, 22.8337) ccw projected
  arc A286 (5.6497, 12.6739) -> (5.72, 13.8624) centre (0.146, 13.5956) ccw projected
  arc A287 (5.72, 13.8624) -> (6.0701, 13.9762) centre (2.9986, 22.8337) ccw projected
  arc A288 (6.0701, 13.9762) -> (6.8255, 13.056) centre (10.7364, 17.0367) ccw projected
  arc A289 (6.8255, 13.056) -> (7.2064, 13.2138) centre (2.9986, 22.8337) ccw projected
  arc A290 (7.2064, 13.2138) -> (7.0899, 14.3986) centre (1.6262, 13.2631) ccw projected
  arc A291 (7.0899, 14.3986) -> (7.4179, 14.5657) centre (2.9986, 22.8337) ccw projected
  arc A292 (7.4179, 14.5657) -> (8.308, 13.775) centre (11.548, 18.3185) ccw projected
  arc A293 (8.308, 13.775) -> (8.6595, 13.9905) centre (2.9986, 22.8337) ccw projected
  arc A294 (8.6595, 13.9905) -> (8.3591, 15.1425) centre (3.1403, 13.1663) ccw projected
  arc A295 (8.3591, 15.1425) -> (8.6569, 15.3589) centre (2.9986, 22.8337) ccw projected
  arc A296 (8.6569, 15.3589) -> (9.6597, 14.7171) centre (12.1491, 19.7115) ccw projected
  arc A297 (9.6597, 14.7171) -> (9.9732, 14.9849) centre (2.9986, 22.8337) ccw projected
  arc A298 (9.9732, 14.9849) -> (9.4963, 16.0757) centre (4.6509, 13.3075) ccw projected
  arc A299 (9.4963, 16.0757) -> (9.7566, 16.336) centre (2.9986, 22.8337) ccw projected
  arc A300 (9.7566, 16.336) -> (10.8474, 15.8591) centre (12.5248, 21.1814) ccw projected
  arc A301 (10.8474, 15.8591) -> (11.1152, 16.1726) centre (2.9986, 22.8337) ccw projected
  arc A302 (11.1152, 16.1726) -> (10.4734, 17.1754) centre (6.1208, 13.6832) ccw projected
  arc A303 (10.4734, 17.1754) -> (10.6898, 17.4732) centre (2.9986, 22.8337) ccw projected
  arc A304 (10.6898, 17.4732) -> (11.8418, 17.1728) centre (12.666, 22.692) ccw projected
  arc A305 (11.8418, 17.1728) -> (12.0573, 17.5243) centre (2.9986, 22.8337) ccw projected
  arc A306 (12.0573, 17.5243) -> (11.2666, 18.4144) centre (7.5138, 14.2843) ccw projected
  arc A307 (11.2666, 18.4144) -> (11.4337, 18.7424) centre (2.9986, 22.8337) ccw projected
  arc A308 (11.4337, 18.7424) -> (12.6185, 18.6259) centre (12.5692, 24.2061) ccw projected
  arc A309 (12.6185, 18.6259) -> (12.7763, 19.0068) centre (2.9986, 22.8337) ccw projected
  arc A310 (12.7763, 19.0068) -> (11.8561, 19.7622) centre (8.7956, 15.0959) ccw projected
  arc A311 (11.8561, 19.7622) -> (11.9699, 20.1123) centre (2.9986, 22.8337) ccw projected
  arc A312 (11.9699, 20.1123) -> (13.1584, 20.1826) centre (12.2367, 25.6863) ccw projected
  arc A313 (13.1584, 20.1826) -> (13.2546, 20.5835) centre (2.9986, 22.8337) ccw projected
  arc A314 (13.2546, 20.5835) -> (12.2276, 21.1856) centre (9.9347, 16.098) ccw projected
  arc A315 (12.2276, 21.1856) -> (12.2851, 21.5492) centre (2.9986, 22.8337) ccw projected
  arc A316 (12.2851, 21.5492) -> (13.448, 21.8046) centre (11.6767, 27.0964) ccw projected
  arc A317 (13.448, 21.8046) -> (13.4804, 22.2156) centre (2.9986, 22.8337) ccw projected
  arc A318 (13.4804, 22.2156) -> (12.3718, 22.6497) centre (10.903, 17.266) ccw projected
  arc A319 (12.3718, 22.6497) -> (12.3718, 23.0178) centre (2.9986, 22.8337) ccw projected
  arc A320 (12.3718, 23.0178) -> (13.4804, 23.4519) centre (10.903, 28.4015) ccw projected
  arc A321 (13.4804, 23.4519) -> (13.448, 23.8629) centre (2.9986, 22.8337) ccw projected
  circle A322 centre (28.4986, 22.8337) radius 10.5
  circle A323 centre (2.9986, 22.8337) radius 10.5
  circle A324 centre (28.4986, 22.8337) radius 10.9
  circle A325 centre (2.9986, 22.8337) radius 10.9
  line L0 (-10.0014, 0) -> (0, 0) projected
  arc A326 (0, 0) -> (10.1832, 0) centre (5.0916, 5.5748) ccw projected
  line L1 (10.1832, 0) -> (43.7986, 0) projected
  line L2 (43.7986, 0) -> (43.7986, 27.7) projected
  line L3 (43.7986, 27.7) -> (31.8346, 27.7) projected
  line L4 (-10.0014, 27.7) -> (-10.0014, 0) projected
  arc A327 (-0.3375, 27.7) -> (6.3346, 27.7) centre (2.9986, 22.8337) ccw projected
  arc A328 (25.1625, 27.7) -> (31.8346, 27.7) centre (28.4986, 22.8337) ccw projected
  line L5 (25.1625, 27.7) -> (6.3346, 27.7) projected
  line L6 (-0.3375, 27.7) -> (-10.0014, 27.7) projected
  point P0 (12.6185, 27.0416)
  point P1 (12.7763, 26.6607)
  point P2 (38.252, 27.7)
  point P3 (-6.7549, 27.7)
  point P4 (18.7451, 27.7)
  point P5 (12.752, 27.7)
  dimension "d56" = 0.4
  dimension "d57" = 0.4
  constraints: 2 centre point, 2 coincident, 6 other
ref_plane "Work Plane5" through (12.9085, 29.7, -6.4252) normal (0, 1, 0) x (-0.0784591, 0, 0.9969173)
ref_plane "Work Plane6" through (12.9085, 29.7, -6.4252) normal (0, 1, 0) x (-0.0784591, 0, 0.9969173)
extrude "Extrusion12" add sketch "Sketch11" along normal blind 4.2 contours A0 | A160 A159 A158 A157 A156 A155 A154 A153 A152 A151 A150 A149 A148 A147 A146 A145 L5 A328 L3 A91 A90 A89 A88 A87 A86 A85 A84 A83 A82 A81 A80 A79 A78 A77 A76 A75 A74 A73 A72 A71 A70 A69 A68 A67 A66 A65 A64 A63 A62 A61 A60 A59 A58 A57 A56 A55 A54 A53 A52 A51 A50 A49 A48 A47 A46 A45 A44 A43 A42 A41 A40 A39 A38 A37 A36 A35 A34 A33 A32 A31 A30 A29 A28 A27 A26 A25 A24 A23 A22 A21 A20 A19 A18 A17 A16 A15 A14 A13 A12 A11 A10 A9 A8 A7 A6 A5 A4 A3 A2 A1 | A322 A4 A8 A12 A16 A20 A24 A28 A32 A36 A40 A44 A48 A52 A56 A60 A64 A68 A72 A76 A80 A84 A88 L3 A324 L5 A148 A152 A156 A160 | A1 A2 A3 A322 | A322 A157 A158 A159 | A5 A6 A7 A322 | A322 A153 A154 A155 | A9 A10 A11 A322 | A322 A149 A150 A151 | A13 A14 A15 A322 | A322 L5 A145 A146 A147 | L5 A324 L3 A322 A92 A96 A100 A104 A108 A112 A116 A120 A124 A128 A132 A136 A140 A144 | A322 A145 L5 | A17 A18 A19 A322 | A144 A143 A142 A141 A140 A139 A138 A137 A136 A135 A134 A133 A132 A131 A130 A129 A128 A127 A126 A125 A124 A123 A122 A121 A120 A119 A118 A117 A116 A115 A114 A113 A112 A111 A110 A109 A108 A107 A106 A105 A104 A103 A102 A101 A100 A99 A98 A97 A96 A95 A94 A93 A92 A91 L3 A328 L5 A145 | A324 L3 L2 L1 A326 L0 L4 L6 A325 L5 | A322 A141 A142 A143 | L5 A323 A173 A177 A181 A185 A189 A193 A197 A201 A205 A209 A213 A217 A221 A225 L6 A325 | A325 L6 A323 A229 A233 A237 A241 A245 A249 A253 A257 A261 A265 A269 A273 A277 A281 A285 A289 A293 A297 A301 A305 A309 A313 A317 A321 A165 A169 L5 | A21 A22 A23 A322 | L3 A91 A322 | A322 A89 A90 A91 L3 | L5 A172 A323 | A323 A170 A171 A172 L5 | A322 A137 A138 A139 | L6 A226 A227 A228 A323 | A323 A226 L6 | A169 A168 A167 A166 A165 A164 A163 A162 A321 A320 A319 A318 A317 A316 A315 A314 A313 A312 A311 A310 A309 A308 A307 A306 A305 A304 A303 A302 A301 A300 A299 A298 A297 A296 A295 A294 A293 A292 A291 A290 A289 A288 A287 A286 A285 A284 A283 A282 A281 A280 A279 A278 A277 A276 A275 A274 A273 A272 A271 A270 A269 A268 A267 A266 A265 A264 A263 A262 A261 A260 A259 A258 A257 A256 A255 A254 A253 A252 A251 A250 A249 A248 A247 A246 A245 A244 A243 A242 A241 A240 A239 A238 A237 A236 A235 A234 A233 A232 A231 A230 A229 A228 A227 A226 L6 A327 L5 A172 A171 A170 | A172 L5 A327 L6 A226 A225 A224 A223 A222 A221 A220 A219 A218 A217 A216 A215 A214 A213 A212 A211 A210 A209 A208 A207 A206 A205 A204 A203 A202 A201 A200 A199 A198 A197 A196 A195 A194 A193 A192 A191 A190 A189 A188 A187 A186 A185 A184 A183 A182 A181 A180 A179 A178 A177 A176 A175 A174 A173 | A25 A26 A27 A322 | A322 A85 A86 A87 | A93 A94 A95 A322 | A323 A166 A167 A168 | A174 A175 A176 A323 | A322 A133 A134 A135 | A323 A222 A223 A224 | A230 A231 A232 A323 | A29 A30 A31 A322 | A322 A81 A82 A83 | A97 A98 A99 A322 | A323 A162 A163 A164 | A178 A179 A180 A323 | A322 A129 A130 A131 | A323 A218 A219 A220 | A234 A235 A236 A323 | A33 A34 A35 A322 | A322 A77 A78 A79 | A101 A102 A103 A322 | A323 A318 A319 A320 | A182 A183 A184 A323 | A322 A125 A126 A127 | A323 A214 A215 A216 | A238 A239 A240 A323 | A37 A38 A39 A322 | A105 A106 A107 A322 | A186 A187 A188 A323 | A322 A121 A122 A123 | A322 A73 A74 A75 | A323 A210 A211 A212 | A242 A243 A244 A323 | A323 A314 A315 A316 | A41 A42 A43 A322 | A109 A110 A111 A322 | A190 A191 A192 A323 | A322 A117 A118 A119 | A322 A69 A70 A71 | A323 A206 A207 A208 | A246 A247 A248 A323 | A323 A310 A311 A312 | A45 A46 A47 A322 | A113 A114 A115 A322 | A194 A195 A196 A323 | A322 A65 A66 A67 | A323 A202 A203 A204 | A250 A251 A252 A323 | A323 A306 A307 A308 | A49 A50 A51 A322 | A198 A199 A200 A323 | A322 A61 A62 A63 | A254 A255 A256 A323 | A323 A302 A303 A304 | A53 A54 A55 A322 | A322 A57 A58 A59 | A258 A259 A260 A323 | A323 A298 A299 A300 | A262 A263 A264 A323 | A323 A294 A295 A296 | A266 A267 A268 A323 | A323 A290 A291 A292 | A270 A271 A272 A323 | A323 A286 A287 A288 | A274 A275 A276 A323 | A323 A282 A283 A284 | A278 A279 A280 A323 | A161
sketch "Sketch13" plane through (-4.2986, 26.6, 27.7) normal (0, 1, 0) x (1, 0, 0)
  circle A0 centre (-3.336, 19.5782) radius 1.0564 projected
  circle A1 centre (-3.336, 19.5782) radius 3
  point P0 (4.2986, 27.7)
  dimension "d65" = 6
  constraints: 2 coincident, 1 centre point
  measures "d65" diameter of A1
extrude "Extrusion14" cut sketch "Sketch13" against normal up to surface (1 mm away) contours A0 | A1
sketch "Sketch14" plane through (-4.2986, 25.6, 27.7) normal (0, 1, 0) x (1, 0, 0)
  circle A0 centre (-3.336, 19.5782) radius 1.0564 projected
  point P0 (4.2986, 27.7)
hole "Hole1" [suppressed]
sketch "Sketch15" plane through (-4.2986, 19.3, 27.7) normal (0, 1, 0) x (1, 0, 0)
  circle A0 centre (7.8331, 8.1218) radius 1.0564 projected
  circle A1 centre (7.8331, 8.1218) radius 2.25
  point P0 (4.2986, 27.7)
  dimension "d75" = 4.5
  constraints: 1 centre point, 1 coincident
  measures "d75" diameter of A1
hole "Hole2" at (3.5346, 19.3, 19.5782) direction (0, -1, 0) diameter 3.1 end through all counterbore diameter 4.5 counterbore depth 2.6 clearance for "Countersunk Flat Head Screw ISO 2009/7046" size "M2.5" standard "ISO"
ref_plane "Work Plane8" through (-2.05, 17.3, 13.85) normal (0, -1, 0) x (0.7160287, 0, -0.6980708)
sketch "Sketch16" plane through (-2.05, 17.3, 13.85) normal (0, -1, 0) x (0.7160287, 0, -0.6980708)
  circle A0 centre (12.3441, 6.6773) radius 1.25 projected
  circle A1 centre (3.9412, 12.0987) radius 1.25 projected
  circle A2 centre (-3.741, 7.91) radius 1.25 projected
  circle A3 centre (-3.741, 7.91) radius 1.55
  circle A4 centre (3.9412, 12.0987) radius 1.55
  circle A5 centre (12.3441, 6.6773) radius 1.55
  point P0 (11.1361, -8.486)
  dimension "d83" = 0.3
  dimension "d84" = 0.3
  dimension "d85" = 0.3
  constraints: 3 centre point
  measures "d83" radial gap between concentric circles of A2 A3
  measures "d84" radial gap between concentric circles of A1 A4
  measures "d85" radial gap between concentric circles of A0 A5
extrude "Extrusion15" cut sketch "Sketch16" against normal through all contours A1 | A2 | A3 | A4
sketch "Sketch17" plane through (-4.2986, 24.5, 27.7) normal (0, 1, 0) x (1, 0, 0)
  circle A0 centre (15.7486, 17.6859) radius 1.25 projected
  circle A1 centre (15.7486, 17.6859) radius 1.55
  point P0 (4.2986, 27.7)
  dimension "d89" = 0.3
  constraints: 1 centre point
  measures "d89" radial gap between concentric circles of A0 A1
extrude "Extrusion16" cut sketch "Sketch17" against normal blind 2 contours A0 | A1
sketch "Sketch18" plane through (19.4905, 16.2, 0) normal (0, 0, -1) x (-1, 0, 0)
  line L0 (0, 0) -> (8.0905, 0) projected
  line L1 (16.4405, 8.3) -> (-0.3595, 8.3) projected
  line L2 (3.6152, 8.3) -> (16.0126, 8.3) projected
  line L3 (8.0905, 8.3) -> (8.0905, 0)
  circle A0 centre (11.3405, 4.15) radius 3.25
  line L4 (14.8905, 9.4) -> (26.6905, 9.4) projected
  line L5 (0, 0) -> (33.7905, 0) projected
  line L6 (33.7905, 9.4) -> (33.7905, 0)
  line L7 (33.7905, 0) -> (23.789, 0) projected
  line L8 (24.1265, 10.4) -> (24.1265, 9.4) projected
  line L9 (14.8905, 9.4) -> (14.8905, 0)
  line L10 (16.1405, 0) -> (26.9405, 0) projected
  line L11 (33.7905, 9.4) -> (14.8905, 0)
  line L12 (33.7905, 0) -> (14.8905, 9.4)
  line L13 (24.7351, 9.4) -> (26.6834, 9.4) projected
  line L14 (33.7905, 9.4) -> (26.6834, 9.4)
  point P0 (19.4905, -16.2)
  point P1 (16.1846, 8.3)
  point P2 (26.087, 9.4)
  point P3 (24.3619, 0)
  point P4 (24.3516, 0)
  point P5 (24.3405, 4.7)
  point P6 (8.0405, 8.3)
  dimension "d92" = 6.5
  dimension "d93" = 4.15
  dimension "d94" = 4.15
  constraints: 12 end point, 3 perpendicular, 2 midpoint, 2 point on line, 1 centre point, 1 coincident, 1 collinear, 1 tangent
  measures "d92" diameter of A0
  measures "d93" vertical distance of A0.centre point (8.04, 8.3)
  measures "d94" vertical distance of L0.end A0.centre
hole "Hole3" at (-4.85, 20.9, 0) at (8.15, 20.35, 0) direction (0, 0, 1) diameter 4 depth 6 counterbore diameter 5 counterbore depth 1
sketch "Sketch19" plane through (-14.3, 16.2, 0) normal (-1, 0, 0) x (0, 0, 1)
  line L0 (18.2328, 3.1) -> (18.2328, 5.7) projected
  line L1 (27.7, 0) -> (27.7, 5.7) projected
  line L2 (0, 0) -> (27.7, 0) projected
  line L3 (18.2328, 3.1) -> (18.2328, 0)
  line L4 (21.1282, 0) -> (18.0282, 0) projected
  line L5 (18.2328, 0) -> (27.7, 13.6)
  line L6 (27.7, 0) -> (18.2328, 13.6)
  point P0 (0, -16.2)
  point P1 (22.9664, 6.8)
  point P2 (18.2328, 8.3)
  point P3 (27.7, 10.4)
  constraints: 6 end point, 1 midpoint, 1 perpendicular, 1 point on line
hole "Hole4" at (-14.3, 23, 22.9664) direction (1, 0, 0) diameter 4 depth 6.5 counterbore diameter 5 counterbore depth 1.5